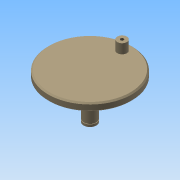
# Autodesk Inventor part: 刀轴带动盘
Saved by Autodesk Inventor 2015 (Build 190159000, 159)
## iProperties
Created: 2017-05-26
Part Number: 刀轴带动盘
Material: 常规
Document SubType Name: Modeling
Designer: Administrator
Density: 1 g/cm^3
Appearance: 麦色
Author: Administrator
Autodesk Inventor part; units mm, degrees
ref_plane "YZ Plane" through (0, 0, 0) normal (1, 0, 0) x (0, 1, 0)
ref_plane "XZ Plane" through (0, 0, 0) normal (0, 1, 0) x (-1, 0, 0)
ref_plane "XY Plane" through (0, 0, 0) normal (0, 0, 1) x (1, 0, 0)
sketch "草图1" plane through (0, 0, 0) normal (0, 0, 1) x (1, 0, 0)
  circle A0 centre (0, 0) radius 65
  dimension "d0" = 130
  constraints: 1 centre point, 1 coincident
  measures "d0" diameter of A0
extrude "拉伸1" add sketch "草图1" along normal blind 12
sketch "草图2" plane through (0, 0, 12) normal (0, 0, 1) x (1, 0, 0)
  circle A0 centre (0, 0) radius 50
  circle A1 centre (0, 50) radius 7.5
  line L0 (0, 0) -> (0, 11.3897)
  dimension "d3" = 100
  dimension "d4" = 15
  dimension "d5" = 11.3897
  constraints: 2 end point, 1 centre point, 1 coincident, 1 point on line, 1 vertical, 1 vertical alignment, 2 other
  measures "d4" diameter of A1
  measures "d5" distance of L0.start L0.end
extrude "拉伸2" add sketch "草图2" along normal blind 15 contours A1 A0 | A0 A1 picked at (0, 47.4583) picked at (0.2152, 52.449)
sketch "草图3" plane through (0, 50, 27) normal (0, 0, 1) x (1, 0, 0)
  circle A0 centre (0, 0) radius 2.5
  circle A1 centre (0, 0) radius 7.5 projected
  point P0 (0, -50)
  dimension "d8" = 5
  constraints: 1 centre point, 1 concentric
  measures "d8" diameter of A0
extrude "拉伸3" cut sketch "草图3" against normal through all contours A0
thread "螺纹1" size "M5x0.8" class "6H" standard "ANSI Metric M Profile" full length
sketch "草图4" plane through (0, 0, 0) normal (0, 0, -1) x (-1, 0, 0)
  circle A0 centre (0, 0) radius 10
  dimension "d13" = 20
  constraints: 1 centre point, 1 coincident
  measures "d13" diameter of A0
extrude "拉伸4" add sketch "草图4" along normal blind 59.7
sketch "草图5" plane through (0, 0, 0) normal (0, 0, -1) x (-1, 0, 0)
  circle A0 centre (0, 0) radius 13
  dimension "d16" = 26
  constraints: 1 centre point, 1 coincident
  measures "d16" diameter of A0
extrude "拉伸5" add sketch "草图5" along normal blind 3
chamfer "倒角1" distance 2 angle 45 2 edges at (-65, 0, 0) (-65, 0, 12)
chamfer "倒角2" distance 0.5 angle 45 1 edges at (10, 0, -59.7)
sketch "草图6" plane through (0, 0, 0) normal (0, 1, 0) x (-1, 0, 0)
  line L0 (-9.175, -54.5) -> (-18.451, -54.5)
  line L1 (-18.451, -54.5) -> (-18.451, -55.7)
  line L2 (-18.451, -55.7) -> (-9.175, -55.7)
  line L3 (-9.175, -55.7) -> (-9.175, -54.5)
  line L4 (9.5, -59.7) -> (-9.5, -59.7) projected
  line L5 (0, -59.7) -> (0, -69.9932)
  point P0 (0, 0)
  dimension "d25" = 10.2932
  dimension "d26" = 4
  dimension "d27" = 1.2
  dimension "d28" = 9.175
  dimension "d29" = 9.276
  constraints: 10 end point, 2 parallel, 1 horizontal, 1 midpoint, 1 perpendicular, 1 vertical
  measures "d25" distance of L5.start L5.end
  measures "d26" distance between parallel lines of L4 L2
  measures "d27" distance of L0.end L1.end
  measures "d28" distance between parallel lines of L5 L3
  measures "d29" distance of L0.start L0.end
revolve "旋转1" cut sketch "草图6" angle 360 about axis through (0, 0, -59.7) along (0, 0, -1)
